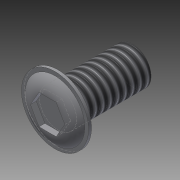
# Autodesk Inventor part: 8020_10series_0.5in_0.25-20_capscrews
Saved by Autodesk Inventor 2014 (Build 180170000, 170)
## iProperties
Created: 2014-10-05
Part Number: 8020_10series_0.5in_0.25-20_capscrews
Material: Generic
Document SubType Name: Modeling
Designer: Matthew
Density: 1 g/cm^3
Appearance: Default
Author: Matthew
Autodesk Inventor part; units mm, degrees
ref_plane "YZ Plane" through (0, 0, 0) normal (1, 0, 0) x (0, 1, 0)
ref_plane "XZ Plane" through (0, 0, 0) normal (0, 1, 0) x (-1, 0, 0)
ref_plane "XY Plane" through (0, 0, 0) normal (0, 0, 1) x (1, 0, 0)
sketch "Sketch1" plane through (0, 0, 0) normal (0, 0, 1) x (1, 0, 0)
  circle A0 centre (0, 0) radius 5.715
  dimension "d0" = 11.43
  constraints: 1 centre point, 1 coincident
  measures "d0" diameter of A0
extrude "Extrusion1" add sketch "Sketch1" along normal blind 0.508
sketch "Sketch2" plane through (0, 0, 0.508) normal (0, 0, 1) x (1, 0, 0)
  circle A0 centre (0, 0) radius 5.715 projected
  circle A1 centre (0, 0) radius 5.08
  dimension "d3" = 10.16
  constraints: 1 centre point, 1 coincident
  measures "d3" diameter of A1
extrude "Extrusion2" add sketch "Sketch2" along normal blind 1.27 contours A1
fillet "Fillet1" radius 3.175 1 edges at (-5.08, 0, 1.778)
sketch "Sketch3" plane through (0, 0, 1.778) normal (0, 0, 1) x (1, 0, 0)
  circle A0 centre (0, 0) radius 2.54 projected
  line L0 (2.9329, 0) -> (1.4665, -2.54)
  line L1 (1.4665, -2.54) -> (-1.4665, -2.54)
  line L2 (-1.4665, -2.54) -> (-2.9329, 0)
  line L3 (-2.9329, 0) -> (-1.4665, 2.54)
  line L4 (-1.4665, 2.54) -> (1.4665, 2.54)
  line L5 (1.4665, 2.54) -> (2.9329, 0)
  dimension "d7" = 2.54
  constraints: 12 end point, 1 coincident, 13 other
  measures "d7" distance from line of point (0, 0) L4
extrude "Extrusion3" cut sketch "Sketch3" against normal blind 1.016
sketch "Sketch4" plane through (0, 0, 0) normal (0, 0, -1) x (-1, 0, 0)
  circle A0 centre (0, 0) radius 5.715 projected
  circle A1 centre (0, 0) radius 3.175
  dimension "d10" = 6.35
  constraints: 1 centre point, 1 coincident
  measures "d10" diameter of A1
extrude "Extrusion4" add sketch "Sketch4" along normal blind 12.7 contours A1
thread "Thread1" size "1/4-20 UNC" class "2A" standard "ANSI Unified Screw Threads" full length
body "Solid1"
